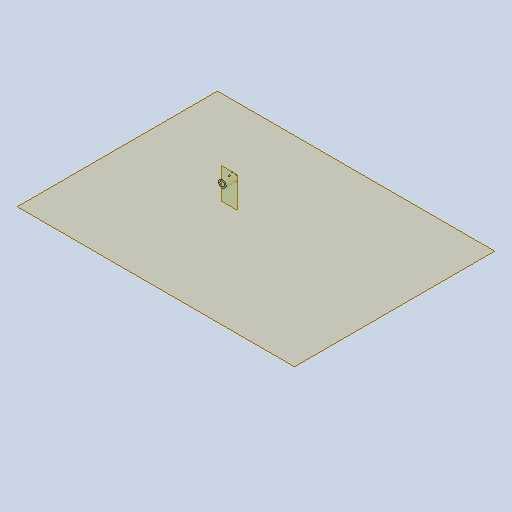
# Autodesk Inventor part: стопорное почти кольцо
Saved by Autodesk Inventor 2024.2 (Build 282272000, 272)
## iProperties
Created: 2025-11-25
Part Number: стопорное почти кольцо
Material: Типовые
Document SubType Name: Modeling
Designer: katya_notebook
Density: 1 g/cm^3
Appearance: По умолчанию
Author: katya_notebook
Autodesk Inventor part; units mm, degrees
ref_plane "YZ Plane" through (0, 0, 0) normal (1, 0, 0) x (0, 1, 0)
ref_plane "XZ Plane" through (0, 0, 0) normal (0, 1, 0) x (-1, 0, 0)
ref_plane "XY Plane" through (0, 0, 0) normal (0, 0, 1) x (1, 0, 0)
ref_plane "РабПлоскость1" through (-501.6702, 157.3163, -333.8297) normal (0, 0, -1) x (0, -1, 0)
sketch "Эскиз1" plane through (-501.6702, 157.3163, -333.8297) normal (0, 0, -1) x (0, -1, 0)
  arc A0 (-15, 7.5) -> (15, 7.5) centre (0, 7.5) ccw projected
  arc A1 (-7.1, 7.5) -> (7.1, 7.5) centre (0, 7.5) ccw projected
  circle A2 centre (0, 7.5) radius 2.5 projected
  circle A3 centre (0, 7.5) radius 2.6
  circle A4 centre (0, 7.5) radius 4
  point P0 (157.3164, -501.6702)
  dimension "d0" = 5.2
  dimension "d1" = 8
  constraints: 2 centre point, 2 coincident
  measures "d0" diameter of A3
  measures "d1" diameter of A4
extrude "Выдавливание1" add sketch "Эскиз1" along normal blind 12.5 contours A4
ref_plane "РабПлоскость2" through (-415.5869, 191.0213, -276.3296) normal (0, 1, 0) x (-1, 0, 0)
sketch "Эскиз2" plane through (-415.5869, 191.0213, -276.3296) normal (0, 1, 0) x (-1, 0, 0)
  circle A0 centre (93.5834, -65) radius 1
  ellipse E0 centre (93.5834, -70) end of major axis (97.5834, -70) minor radius 0 projected
  line L0 (89.5834, -57.5) -> (89.5834, -70) projected
  point P0 (-415.5869, 276.3296)
  dimension "d4" = 2
  dimension "d5" = 5
  dimension "d6" = 4
  constraints: 1 centre point, 1 horizontal alignment
  measures "d4" diameter of A0
  measures "d5" distance of point (93.583, -70) A0.centre
  measures "d6" distance from line of L0 A0.centre
extrude "Выдавливание2" cut sketch "Эскиз2" against normal blind 61.25
